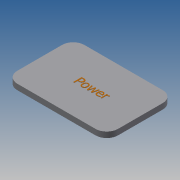
# Autodesk Inventor part: pullbox
Saved by Autodesk Inventor 2014 SP1 (Build 180222100, 222)
## iProperties
Created: 2014-12-12
Part Number: pullbox
Material: Generic
Document SubType Name: Modeling
Designer: Dave
Density: 1 g/cm^3
Appearance: Default
Author: Dave
Autodesk Inventor part; units mm, degrees
ref_plane "YZ Plane" through (0, 0, 0) normal (1, 0, 0) x (0, 1, 0)
ref_plane "XZ Plane" through (0, 0, 0) normal (0, 1, 0) x (-1, 0, 0)
ref_plane "XY Plane" through (0, 0, 0) normal (0, 0, 1) x (1, 0, 0)
sketch "Sketch1" plane through (0, 0, 0) normal (0, 1, 0) x (-1, 0, 0)
  line L0 (101.6, 0) -> (812.8, 0)
  line L1 (914.4, 101.6) -> (914.4, 508)
  line L2 (812.8, 609.6) -> (101.6, 609.6)
  line L3 (0, 508) -> (0, 101.6)
  arc A0 (101.6, 609.6) -> (0, 508) centre (101.6, 508) ccw
  arc A1 (0, 101.6) -> (101.6, 0) centre (101.6, 101.6) ccw
  arc A2 (812.8, 0) -> (914.4, 101.6) centre (812.8, 101.6) ccw
  arc A3 (914.4, 508) -> (812.8, 609.6) centre (812.8, 508) ccw
  point P0 (0, 0)
  point P1 (914.4, 609.6)
  point P2 (914.4, 0)
  point P3 (0, 609.6)
  dimension "d0" = 914.4
  dimension "d1" = 609.6
  dimension "d9" = 101.6
  constraints: 8 end point, 8 point on circle, 8 point on line, 8 tangent, 4 centre point, 3 equal radius, 2 parallel, 1 horizontal, 1 perpendicular
  measures "d0" distance of point (0, 609.6) point (914.4, 609.6)
  measures "d1" distance of point (914.4, 609.6) point (914.4, 0)
  measures "d9" radius of A0
extrude "Extrusion1" add sketch "Sketch1" along normal blind 50.8
sketch "Sketch8" plane through (0, 50.8, 0) normal (0, 1, 0) x (1, 0, 0)
  line L0 (-577.5208, -267.3319) -> (-568.3422, -267.3319) construction
  line L1 (-568.3422, -267.3319) -> (-568.3422, -270.58) construction
  line L2 (-568.3422, -270.58) -> (-577.5208, -270.58) construction
  line L3 (-577.5208, -270.58) -> (-577.5208, -267.3319) construction
  spline S0 degree 2 poles (-521.6367, -290.3031) (-521.6367, -295.2431) (-525.1565, -304.1352) (-528.3057, -307.2227) knots 0 0 0 1 2 2 2
  spline S1 degree 2 poles (-528.3057, -307.2227) (-532.2577, -311.113) (-542.9406, -315.1268) (-551.0916, -315.1268) knots 0 0 0 1 2 2 2
  line L4 (-551.0916, -315.1268) -> (-559.6749, -315.1268)
  line L5 (-559.6749, -315.1268) -> (-559.6749, -343.5319)
  line L6 (-559.6749, -343.5319) -> (-569.802, -343.5319)
  line L7 (-569.802, -343.5319) -> (-569.802, -267.3319)
  line L8 (-569.802, -267.3319) -> (-550.6594, -267.3319)
  spline S2 degree 2 poles (-550.6594, -267.3319) (-543.8668, -267.3319) (-534.3573, -269.555) (-530.714, -272.0867) knots 0 0 0 1 2 2 2
  spline S3 degree 2 poles (-530.714, -272.0867) (-526.4532, -274.989) (-521.6367, -283.9428) (-521.6367, -290.3031) knots 0 0 0 1 2 2 2
  spline S4 degree 2 poles (-532.196, -290.6118) (-532.196, -286.6598) (-534.913, -280.8553) (-537.6918, -279.0028) knots 0 0 0 1 2 2 2
  spline S5 degree 2 poles (-537.6918, -279.0028) (-540.1001, -277.3973) (-546.5221, -276.1005) (-551.2769, -276.1005) knots 0 0 0 1 2 2 2
  line L9 (-551.2769, -276.1005) -> (-559.6749, -276.1005)
  line L10 (-559.6749, -276.1005) -> (-559.6749, -306.4817)
  line L11 (-559.6749, -306.4817) -> (-552.7589, -306.4817)
  spline S6 degree 2 poles (-552.7589, -306.4817) (-546.5838, -306.4817) (-538.9885, -304.5057) (-536.5185, -301.9122) knots 0 0 0 1 2 2 2
  spline S7 degree 2 poles (-536.5185, -301.9122) (-534.2338, -299.6274) (-532.196, -294.2551) (-532.196, -290.6118) knots 0 0 0 1 2 2 2
  spline S8 degree 2 poles (-465.7526, -314.9415) (-465.7526, -329.3911) (-479.6464, -345.1374) (-491.2555, -345.1374) knots 0 0 0 1 2 2 2
  spline S9 degree 2 poles (-491.2555, -345.1374) (-503.1733, -345.1374) (-516.8201, -328.8971) (-516.8201, -314.9415) knots 0 0 0 1 2 2 2
  spline S10 degree 2 poles (-516.8201, -314.9415) (-516.8201, -300.6154) (-502.7411, -284.7456) (-491.2555, -284.7456) knots 0 0 0 1 2 2 2
  spline S11 degree 2 poles (-491.2555, -284.7456) (-479.6464, -284.7456) (-465.7526, -300.5537) (-465.7526, -314.9415) knots 0 0 0 1 2 2 2
  spline S12 degree 2 poles (-475.6944, -314.9415) (-475.6944, -303.8264) (-483.7837, -293.0201) (-491.2555, -293.0201) knots 0 0 0 1 2 2 2
  spline S13 degree 2 poles (-491.2555, -293.0201) (-498.7273, -293.0201) (-506.8783, -303.8264) (-506.8783, -314.9415) knots 0 0 0 1 2 2 2
  spline S14 degree 2 poles (-506.8783, -314.9415) (-506.8783, -325.7478) (-498.7273, -336.8629) (-491.2555, -336.8629) knots 0 0 0 1 2 2 2
  spline S15 degree 2 poles (-491.2555, -336.8629) (-483.8454, -336.8629) (-475.6944, -325.9331) (-475.6944, -314.9415) knots 0 0 0 1 2 2 2
  line L12 (-386.5885, -286.3511) -> (-401.0999, -343.5319)
  line L13 (-401.0999, -343.5319) -> (-409.9919, -343.5319)
  line L14 (-409.9919, -343.5319) -> (-423.9475, -299.4421)
  line L15 (-423.9475, -299.4421) -> (-437.8414, -343.5319)
  line L16 (-437.8414, -343.5319) -> (-446.6717, -343.5319)
  line L17 (-446.6717, -343.5319) -> (-461.3065, -286.3511)
  line L18 (-461.3065, -286.3511) -> (-451.303, -286.3511)
  line L19 (-451.303, -286.3511) -> (-441.1759, -330.6261)
  line L20 (-441.1759, -330.6261) -> (-427.6526, -286.3511)
  line L21 (-427.6526, -286.3511) -> (-419.6868, -286.3511)
  line L22 (-419.6868, -286.3511) -> (-405.7929, -330.6261)
  line L23 (-405.7929, -330.6261) -> (-396.2834, -286.3511)
  line L24 (-396.2834, -286.3511) -> (-386.5885, -286.3511)
  spline S16 degree 2 poles (-353.3051, -344.8287) (-367.0137, -344.8287) (-382.0808, -329.4528) (-382.0808, -315.2503) knots 0 0 0 1 2 2 2
  spline S17 degree 2 poles (-382.0808, -315.2503) (-382.0808, -301.2947) (-367.4459, -284.7456) (-355.6516, -284.7456) knots 0 0 0 1 2 2 2
  spline S18 degree 2 poles (-355.6516, -284.7456) (-350.3411, -284.7456) (-342.1283, -287.8331) (-339.1025, -291.1058) knots 0 0 0 1 2 2 2
  spline S19 degree 2 poles (-339.1025, -291.1058) (-336.015, -294.3786) (-332.7422, -303.8264) (-332.7422, -310.6807) knots 0 0 0 1 2 2 2
  line L25 (-332.7422, -310.6807) -> (-332.7422, -315.9295)
  line L26 (-332.7422, -315.9295) -> (-372.3242, -315.9295)
  spline S20 degree 2 poles (-372.3242, -315.9295) (-372.3242, -325.8713) (-362.3206, -336.4306) (-353.4286, -336.4306) knots 0 0 0 1 2 2 2
  spline S21 degree 2 poles (-353.4286, -336.4306) (-350.2793, -336.4306) (-344.166, -335.0104) (-341.696, -333.8989) knots 0 0 0 1 2 2 2
  spline S22 degree 2 poles (-341.696, -333.8989) (-339.1025, -332.6639) (-335.521, -330.5026) (-334.3477, -329.5146) knots 0 0 0 1 2 2 2
  line L27 (-334.3477, -329.5146) -> (-333.792, -329.5146)
  line L28 (-333.792, -329.5146) -> (-333.792, -340.0122)
  spline S23 degree 2 poles (-333.792, -340.0122) (-335.4592, -340.6914) (-340.5227, -342.6674) (-342.4988, -343.2232) knots 0 0 0 1 2 2 2
  spline S24 degree 2 poles (-342.4988, -343.2232) (-345.2775, -344.0259) (-349.8471, -344.8287) (-353.3051, -344.8287) knots 0 0 0 1 2 2 2
  spline S25 degree 2 poles (-342.1283, -308.5812) (-342.2518, -304.6909) (-343.8573, -299.0099) (-345.401, -297.0956) knots 0 0 0 1 2 2 2
  spline S26 degree 2 poles (-345.401, -297.0956) (-347.0683, -294.9344) (-352.3171, -292.6496) (-356.2073, -292.6496) knots 0 0 0 1 2 2 2
  spline S27 degree 2 poles (-356.2073, -292.6496) (-360.0359, -292.6496) (-365.4082, -294.9344) (-367.6312, -297.1574) knots 0 0 0 1 2 2 2
  spline S28 degree 2 poles (-367.6312, -297.1574) (-369.7924, -299.4421) (-372.0155, -304.9379) (-372.3242, -308.5812) knots 0 0 0 1 2 2 2
  line L29 (-372.3242, -308.5812) -> (-342.1283, -308.5812)
  line L30 (-292.6662, -296.6634) -> (-293.1602, -296.6634)
  spline S29 degree 2 poles (-293.1602, -296.6634) (-294.2717, -296.3546) (-296.68, -296.2311) (-298.3472, -296.2311) knots 0 0 0 1 2 2 2
  spline S30 degree 2 poles (-298.3472, -296.2311) (-302.2375, -296.2311) (-309.8945, -299.6274) (-313.3526, -302.9619) knots 0 0 0 1 2 2 2
  line L31 (-313.3526, -302.9619) -> (-313.3526, -343.5319)
  line L32 (-313.3526, -343.5319) -> (-322.9856, -343.5319)
  line L33 (-322.9856, -343.5319) -> (-322.9856, -286.3511)
  line L34 (-322.9856, -286.3511) -> (-313.3526, -286.3511)
  line L35 (-313.3526, -286.3511) -> (-313.3526, -294.8726)
  spline S31 degree 2 poles (-313.3526, -294.8726) (-308.1038, -290.1796) (-300.2615, -286.3511) (-296.5565, -286.3511) knots 0 0 0 1 2 2 2
  spline S32 degree 2 poles (-296.5565, -286.3511) (-295.0744, -286.3511) (-293.5924, -286.4746) (-292.6662, -286.6598) knots 0 0 0 1 2 2 2
  line L36 (-292.6662, -286.6598) -> (-292.6662, -296.6634)
  point P0 (0, 0)
  constraints: 2 other
emboss "Emboss1" sketch "Sketch8" operation add depth 2.54 direction (0, -1, 0)
body "Solid1"
